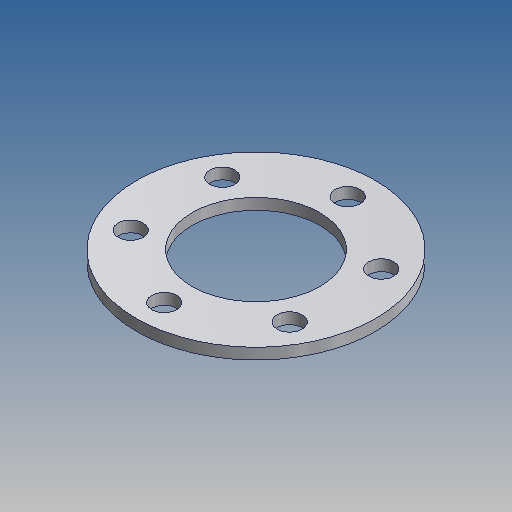
# Autodesk Inventor part: P025
Saved by Autodesk Inventor 2021.4 (Build 254397000, 397)
## iProperties
Company: HES-SO
Created: 2022-06-11
Part Number: P025
Material: Polytetrafluoroethylene
Document SubType Name: Modeling
Designer: HER & ZAE
Density: 2.02 g/cm^3
Appearance: PTFE
Author: HER & ZAE
Title: Joint Carter Arbre
Autodesk Inventor part; units mm, degrees
ref_plane "YZ Plane" through (0, 0, 0) normal (1, 0, 0) x (0, 1, 0)
ref_plane "XZ Plane" through (0, 0, 0) normal (0, 1, 0) x (-1, 0, 0)
ref_plane "XY Plane" through (0, 0, 0) normal (0, 0, 1) x (1, 0, 0)
sketch "Sketch2" plane through (0, 0, 0) normal (0, 0, 1) x (1, 0, 0)
  circle A0 centre (0, 0) radius 11.5
  circle A1 centre (0, 0) radius 21.5
  dimension "d0" = 23
  dimension "d1" = 10
  constraints: 2 centre point, 2 coincident
  measures "d0" diameter of A0
  measures "d1" radial gap between concentric circles of A1 A0
extrude "Extrusion1" add sketch "Sketch2" along normal blind 2
sketch "Sketch3" plane through (0, 0, 2) normal (0, 0, 1) x (1, 0, 0)
  circle A0 centre (0, 0) radius 21.5 construction
  circle A1 centre (0, 0) radius 11.5 construction
  circle A2 centre (0, 0) radius 16.5 construction
  point P0 (0, 16.5)
  point P1 (-14.2894, 8.25)
  point P2 (-14.2894, -8.25)
  point P3 (0, -16.5)
  point P4 (14.2894, -8.25)
  point P5 (14.2894, 8.25)
  dimension "d13" = 33
  dimension "d16" = 360
  constraints: 2 vertical alignment, 1 coincident, 9 other
hole "Hole1" at (-14.2894, 8.25, 2) at (0, 16.5, 2) at (14.2894, 8.25, 2) at (14.2894, -8.25, 2) at (0, -16.5, 2) at (-14.2894, -8.25, 2) direction (0, 0, -1) diameter 4.5 end through all clearance for "Flat Head Machine Screw" size "M4" standard "Ansi Metric M Profile"
body "Solid1"
